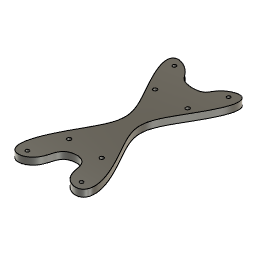
Support carte alim robot v3 v2 (Autodesk Fusion 360 design; units mm, degrees)
Autodesk Fusion 360 part; units mm, degrees
sketch "Esquisse1" plane through (0, 0, 0) normal (0, 0, 1) x (1, 0, 0)
  line L0 (-40, 18) -> (38, 18) construction
  line L1 (38, 18) -> (38, -168) construction
  line L2 (38, -168) -> (-40, -168) construction
  line L3 (-40, -168) -> (-40, 18) construction
  line L4 (-40, 10) -> (38, 10) construction
  line L5 (-32.5, 18) -> (-32.5, -168) construction
  line L6 (30.5, 18) -> (30.5, -168) construction
  line L7 (-40, -161) -> (38, -161) construction
  circle A0 centre (-32.5, 10) radius 2
  circle A1 centre (30.5, 10) radius 2
  circle A2 centre (30.5, -161) radius 2
  circle A3 centre (-32.5, -161) radius 2
  line L8 (-40, -25) -> (38, -25) construction
  line L9 (-40, -125) -> (38, -125) construction
  line L10 (-20, 18) -> (-20, -168) construction
  line L11 (18, 18) -> (18, -168) construction
  circle A4 centre (18, -25) radius 2.25
  circle A5 centre (-20, -25) radius 2.25
  circle A6 centre (18, -125) radius 2.25
  circle A7 centre (-20, -125) radius 2.25
  spline S0 degree 5 poles (-40, 18) (-39.2626, 18.3979) (-37.5852, 18.9177) (-34.537, 18.8921) (-29.8391, 17.4433) (-24.1762, 14.0804) (-19.725, 10.0681) (-16.789, 6.1902) (-14.4925, 2.887) (-11.5565, 0.3626) (-7.0087, -1.3104) (-1.1211, -2.0655) (4.9058, -1.8324) (9.7987, -0.5713) (12.8219, 1.7038) (14.6641, 4.9049) (16.751, 8.8031) (20.3625, 12.9692) (25.6291, 16.6761) (31.6612, 19.0297) (37.157, 19.2002) (40.8171, 16.6008) (41.9256, 11.136) (40.3825, 3.1581) (36.5239, -6.6958) (31.0092, -17.6294) (24.6815, -28.8262) (18.4386, -39.5865) (13.1025, -49.4575) (9.2801, -58.3861) (7.3572, -66.625) (7.5097, -74.6084) (9.709, -82.8407) (13.7281, -91.7759) (19.1508, -101.7086) (25.3713, -112.6432) (31.6207, -124.2229) (37.0825, -135.8568) (40.9927, -146.8155) (42.7471, -156.3379) (42.0036, -163.7329) (38.7912, -168.4856) (33.6071, -170.3567) (27.5443, -169.4962) (21.8997, -166.3523) (17.7374, -161.5654) (15.4829, -155.8693) (14.4633, -149.9862) (13.4191, -144.5838) (11.1011, -140.2346) (6.7888, -137.3761) (0.9629, -136.2658) (-5.143, -136.9838) (-10.2201, -139.4456) (-13.4668, -143.4121) (-15.2533, -148.4988) (-16.6419, -154.2011) (-18.8304, -159.9181) (-22.6683, -164.9806) (-28.029, -168.6673) (-34.0175, -170.2953) (-39.4366, -169.3372) (-43.1406, -165.5189) (-44.4974, -158.9526) (-43.3806, -150.073) (-40.0384, -139.5205) (-35.0038, -128.0415) (-28.9893, -116.3839) (-22.7856, -105.1894) (-17.1643, -94.8992) (-12.7658, -85.6239) (-10.0442, -77.1447) (-9.2737, -69.0538) (-10.538, -60.8593) (-13.7279, -52.1022) (-18.5323, -42.4726) (-24.4378, -31.9156) (-30.7089, -20.7712) (-36.4885, -9.6841) (-40.9308, 0.5497) (-43.3231, 9.1141) (-43.2341, 14.0732) (-42.0096, 16.5306) (-40.7374, 17.6021) (-40, 18) knots 0 0 0 0 0 0 0.0125 0.025 0.0375 0.05 0.0625 0.075 0.0875 0.1 0.1125 0.125 0.1375 0.15 0.1625 0.175 0.1875 0.2 0.2125 0.225 0.2375 0.25 0.2625 0.275 0.2875 0.3 0.3125 0.325 0.3375 0.35 0.3625 0.375 0.3875 0.4 0.4125 0.425 0.4375 0.45 0.4625 0.475 0.4875 0.5 0.5125 0.525 0.5375 0.55 0.5625 0.575 0.5875 0.6 0.6125 0.625 0.6375 0.65 0.6625 0.675 0.6875 0.7 0.7125 0.725 0.7375 0.75 0.7625 0.775 0.7875 0.8 0.8125 0.825 0.8375 0.85 0.8625 0.875 0.8875 0.9 0.9125 0.925 0.9375 0.95 0.9625 0.975 0.9875 1 1 1 1 1 1
  point P0 (-20, 10)
  point P1 (-10, 0)
  point P2 (10, 0)
  point P3 (18, 10)
  point P4 (18, -40.5649)
  point P5 (18, -99.5027)
  point P6 (18, -161)
  point P7 (10, -140)
  point P8 (-10, -140)
  point P9 (-20, -161)
  point P10 (-20, -100)
  point P11 (-20, -40)
  dimension "d1" = 78
  dimension "d2" = 186
  dimension "d5" = 8
  dimension "d6" = 7.5
  dimension "d7" = 7.5
  dimension "d8" = 7
  dimension "d9" = 4
  dimension "d10" = 4
  dimension "d11" = 4
  dimension "d12" = 4
  dimension "d13" = 63
  dimension "d14" = 7.5
  dimension "d15" = 7.5
  dimension "d16" = 63
  dimension "d17" = 100
  dimension "d18" = 43
  dimension "d19" = 43
  dimension "d20" = 186
  dimension "d24" = 4.5
  dimension "d25" = 4.5
  dimension "d26" = 4.5
  dimension "d27" = 4.5
  dimension "d30" = 171
  dimension "d32" = 38
  constraint horizontal L0
  constraint vertical L1
  constraint horizontal L2
  constraint vertical L3
  constraint coincident L3 L4.start
  constraint coincident L1 L4.end
  constraint perpendicular L1 L4
  constraint coincident L0 L5.start
  constraint perpendicular L0 L5
  constraint coincident L0 L6.start
  constraint perpendicular L4 L6
  constraint coincident L3 L7.start
  constraint coincident L1 L7.end
  constraint perpendicular L1 L7
  constraint coincident L4 A0.centre
  constraint coincident L5 A0.centre
  constraint coincident L6 A1.centre
  constraint coincident L4 A1.centre
  constraint coincident L7 A2.centre
  constraint coincident L6 A2.centre
  constraint coincident L7 A3.centre
  constraint coincident L5 A3.centre
  constraint coincident L3 L8.start
  constraint coincident L1 L8.end
  constraint perpendicular L1 L8
  constraint coincident L3 L9.start
  constraint coincident L1 L9.end
  constraint perpendicular L1 L9
  constraint coincident L0 L10.start
  constraint perpendicular L0 L10
  constraint coincident L0 L11.start
  constraint perpendicular L8 L11
  constraint coincident L11 A4.centre
  constraint coincident L8 A4.centre
  constraint coincident L10 A5.centre
  constraint coincident L8 A5.centre
  constraint coincident L11 A6.centre
  constraint coincident L9 A6.centre
  constraint coincident L9 A7.centre
  constraint coincident L10 A7.centre
  constraint coincident L4 P0
  constraint coincident L10 P0
  constraint coincident L11 P3
  constraint coincident L4 P3
  constraint coincident L11 P4
  constraint coincident L11 P5
  constraint coincident L7 P6
  constraint coincident L11 P6
  constraint coincident L7 P9
  constraint coincident L10 P9
  constraint coincident L10 P10
  constraint coincident L10 P11
  measures "d1" distance of L0.start L0.end
  measures "d2" distance of L0 L2
  measures "d5" vertical distance of L4.start L5.start
  measures "d6" distance of L0.start L5.start
  measures "d7" distance of L0.end L6.start
  measures "d8" distance of L2.end L7.start
  measures "d9" diameter of A0
  measures "d10" diameter of A1
  measures "d11" diameter of A2
  measures "d12" diameter of A3
  measures "d13" distance of A0.centre A1.centre
  measures "d14" distance of L2.end L5.end
  measures "d15" distance of L1.end L6.end
  measures "d16" distance of A2.centre A3.centre
  measures "d17" distance of L8 L9
  measures "d18" distance of L0 L8
  measures "d19" distance of L2 L9
  measures "d20" distance of L10.start L10.end
  measures "d24" diameter of A4
  measures "d25" diameter of A5
  measures "d26" diameter of A6
  measures "d27" diameter of A7
  measures "d30" distance of A0.centre A3.centre
  measures "d32" distance of A4.centre A5.centre
extrude "Extrusion1" add sketch "Esquisse1" along normal blind 8
named bodies: "support alim"
